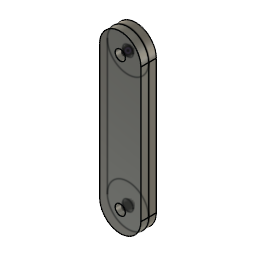
PassiveLink (Autodesk Fusion 360 design; units mm, degrees)
part number: 2026-02-01-17-53-22-850
Autodesk Fusion 360 part; units mm, degrees
sketch "Sketch1" plane through (0, 0, 0) normal (0, 1, 0) x (1, 0, 0)
  circle A0 centre (0, 0) radius 20
  line L0 (-20, 0) -> (-20, 130)
  line L1 (20, 130) -> (20, 0)
  circle A1 centre (0, 130) radius 20
  circle A2 centre (0, 0) radius 5
  circle A3 centre (0, 130) radius 5
  dimension "d1" = 40
  dimension "d3" = 40
  dimension "d5" = 20
  dimension "d6" = 130
  dimension "d9" = 10
  dimension "d10" = 10
  constraint coincident A0.centre A2.centre
  constraint coincident A0 L0.start
  constraint tangent A0 L0
  constraint vertical L0
  constraint coincident A0 L1.end
  constraint tangent A0 L1
  constraint coincident A1 L1.start
  constraint coincident A1 L0.end
  constraint tangent L1 A1
  constraint concentric A0 A2
  constraint concentric A1 A3
  measures "d1" diameter of A0
  measures "d3" diameter of A1
  measures "d5" distance of L0 A1.centre
  measures "d6" distance of L1.end L1.start
  measures "d9" diameter of A2
  measures "d10" diameter of A3
extrude "Extrude1" add sketch "Sketch1" along normal mid plane 15 contours A0 | A0 L0 L1 A1 | A1 | A2 | A3
extrude "Extrude2" cut sketch "Sketch1" along normal through all and the other way through all contours A2 | A3
